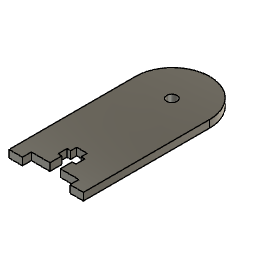
part_A16 (Autodesk Fusion 360 design; units mm, degrees)
Autodesk Fusion 360 part; units mm, degrees
sketch "Sketch1" plane through (0, 0, 0) normal (0, 0, 1) x (1, 0, 0)
  line L0 (0, 0) -> (25, 0)
  line L1 (25, 0) -> (25, 55)
  line L2 (25, 55) -> (0, 55)
  line L3 (0, 55) -> (0, 0)
  dimension "d1" = 25
  dimension "d2" = 55
  constraint horizontal L0
  constraint vertical L1
  constraint horizontal L2
  constraint vertical L3
  constraint coincident L0.start L3.end
  measures "d1" distance of L0.start L0.end
  measures "d2" distance of L0.start L2.end
extrude "Extrude1" add sketch "Sketch1" along normal blind 2.5
sketch "Sketch2" plane through (0, 0, 0) normal (0, -1, 0) x (1, 0, 0)
  line L0 (0, 0) -> (25, 0)
  line L1 (25, 0) -> (25, 2.5)
  line L2 (25, 2.5) -> (0, 2.5)
  line L3 (0, 2.5) -> (0, 0)
  line L4 (0, 2.5) -> (4.5, 2.5)
  line L5 (4.5, 2.5) -> (4.5, 0)
  line L6 (4.5, 0) -> (0, 0)
  line L7 (0, 0) -> (0, 2.5)
  line L8 (25, 2.5) -> (20.5, 2.5)
  line L9 (20.5, 2.5) -> (20.5, 0)
  line L10 (20.5, 0) -> (25, 0)
  line L11 (25, 0) -> (25, 2.5)
  dimension "d5" = 4.5
  dimension "d6" = 4.5
  constraint horizontal L4
  constraint vertical L5
  constraint horizontal L6
  constraint vertical L7
  constraint coincident L2.end L3.start
  constraint horizontal L8
  constraint vertical L9
  constraint horizontal L10
  constraint vertical L11
  constraint coincident L1.end L2.start
  measures "d5" distance of L2.end L4.end
  measures "d6" distance of L1.end L8.end
extrude "Extrude2" cut sketch "Sketch2" against normal blind 3 contours L0 L2 L5 L9
sketch "Sketch3" plane through (0, 3, 0) normal (0, -1, 0) x (1, 0, 0)
  line L0 (4.5, 2.5) -> (4.5, 0)
  line L1 (4.5, 0) -> (20.5, 0)
  line L2 (20.5, 0) -> (20.5, 2.5)
  line L3 (20.5, 2.5) -> (4.5, 2.5)
  line L4 (10.75, 2.5) -> (14.25, 2.5)
  line L5 (14.25, 2.5) -> (14.25, 0)
  line L6 (14.25, 0) -> (10.75, 0)
  line L7 (10.75, 0) -> (10.75, 2.5)
  dimension "d9" = 3.5
  dimension "d10" = 6.25
  constraint horizontal L4
  constraint vertical L5
  constraint horizontal L6
  constraint vertical L7
  constraint coincident L3 L4.start
  measures "d9" distance of L4.start L4.end
  measures "d10" distance of L0 L7
extrude "Extrude3" cut sketch "Sketch3" against normal blind 4 contours L1 L3 L4 L5 L6 L7
sketch "Sketch4" plane through (0, 0, 2.5) normal (0, 0, 1) x (-1, 0, 0)
  line L0 (-10.75, -3) -> (-10.75, -7)
  line L1 (-10.75, -7) -> (-14.25, -7)
  line L2 (-14.25, -7) -> (-14.25, -3)
  line L3 (-14.25, -3) -> (-20.5, -3)
  line L4 (-20.5, -3) -> (-20.5, 0)
  line L5 (-20.5, 0) -> (-25, 0)
  line L6 (-25, 0) -> (-25, -55)
  line L7 (-25, -55) -> (0, -55)
  line L8 (0, -55) -> (0, 0)
  line L9 (0, 0) -> (-4.5, 0)
  line L10 (-4.5, 0) -> (-4.5, -3)
  line L11 (-4.5, -3) -> (-10.75, -3)
  line L12 (-9.5, -7) -> (-15.5, -7)
  line L13 (-15.5, -7) -> (-15.5, -10)
  line L14 (-15.5, -10) -> (-9.5, -10)
  line L15 (-9.5, -10) -> (-9.5, -7)
  dimension "d13" = 6
  dimension "d14" = 3
  dimension "d15" = 1.25
  constraint horizontal L12
  constraint vertical L13
  constraint horizontal L14
  constraint vertical L15
  measures "d13" distance of L12.start L12.end
  measures "d14" distance of L12.start L14.end
  measures "d15" distance of L0 L15
extrude "Extrude4" cut sketch "Sketch4" against normal blind 3 contours L1 L12 L13 L14 L15
sketch "Sketch5" plane through (0, 10, 0) normal (0, -1, 0) x (1, 0, 0)
  line L0 (9.5, 0) -> (15.5, 0)
  line L1 (15.5, 0) -> (15.5, 2.5)
  line L2 (15.5, 2.5) -> (9.5, 2.5)
  line L3 (9.5, 2.5) -> (9.5, 0)
  line L4 (10.75, 2.5) -> (14.25, 2.5)
  line L5 (14.25, 2.5) -> (14.25, 0)
  line L6 (14.25, 0) -> (10.75, 0)
  line L7 (10.75, 0) -> (10.75, 2.5)
  dimension "d18" = 3.5
  dimension "d19" = 2.5
  dimension "d20" = 1.25
  constraint horizontal L4
  constraint vertical L5
  constraint horizontal L6
  constraint vertical L7
  constraint coincident L2 L4.start
  measures "d18" distance of L4.start L4.end
  measures "d19" distance of L4.start L6.end
  measures "d20" distance of L3 L7
extrude "Extrude5" cut sketch "Sketch5" against normal blind 2 contours L0 L2 L4 L5 L6 L7
sketch "Sketch6" plane through (0, 0, 2.5) normal (0, 0, 1) x (-1, 0, 0)
  line L0 (-10.75, -10) -> (-10.75, -12)
  line L1 (-10.75, -12) -> (-14.25, -12)
  line L2 (-14.25, -12) -> (-14.25, -10)
  line L3 (-14.25, -10) -> (-15.5, -10)
  line L4 (-15.5, -10) -> (-15.5, -7)
  line L5 (-15.5, -7) -> (-14.25, -7)
  line L6 (-14.25, -7) -> (-14.25, -3)
  line L7 (-14.25, -3) -> (-20.5, -3)
  line L8 (-20.5, -3) -> (-20.5, 0)
  line L9 (-20.5, 0) -> (-25, 0)
  line L10 (-25, 0) -> (-25, -55)
  line L11 (-25, -55) -> (0, -55)
  line L12 (0, -55) -> (0, 0)
  line L13 (0, 0) -> (-4.5, 0)
  line L14 (-4.5, 0) -> (-4.5, -3)
  line L15 (-4.5, -3) -> (-10.75, -3)
  line L16 (-10.75, -3) -> (-10.75, -7)
  line L17 (-10.75, -7) -> (-9.5, -7)
  line L18 (-9.5, -7) -> (-9.5, -10)
  line L19 (-9.5, -10) -> (-10.75, -10)
  circle A0 centre (-12.5, -42.25) radius 1.75
  dimension "d23" = 3.5
  dimension "d24" = 12.75
  measures "d23" diameter of A0
  measures "d24" distance of L11 A0.centre
extrude "Extrude6" cut sketch "Sketch6" against normal blind 3 contours A0
fillet "Fillet1" radius 12.5 1 edges at (25, 55, 1.25)
fillet "Fillet2" radius 12.5 1 edges at (0, 55, 1.25)
